Autodesk Inventor part; units mm, degrees
(part 2 of 2)
sketch "PCB草图" plane through (0, 3.5, 0) normal (0, 1, 0) x (1, 0, 0)
  line L0 (-85.025, -120.975) -> (-85.025, -135.025) projected
  line L1 (-85.025, -135.025) -> (-70.975, -135.025) projected
  line L2 (-70.975, -120.975) -> (-85.025, -120.975) projected
  line L3 (-70.975, -135.025) -> (-70.975, -120.975) projected
  line L4 (-85.025, -135.025) -> (-70.975, -120.975) construction
  line L5 (-70.975, -135.025) -> (-85.025, -120.975) construction
  line L6 (-85.025, -116.025) -> (-70.975, -116.025) projected
  line L7 (-85.025, -101.975) -> (-85.025, -116.025) projected
  line L8 (-70.975, -101.975) -> (-85.025, -101.975) projected
  line L9 (-70.975, -116.025) -> (-70.975, -101.975) projected
  line L10 (-85.025, -116.025) -> (-70.975, -101.975) construction
  line L11 (-70.975, -116.025) -> (-85.025, -101.975) construction
  line L12 (-85.025, -82.975) -> (-85.025, -97.025) projected
  line L13 (-85.025, -97.025) -> (-70.975, -97.025) projected
  line L14 (-70.975, -97.025) -> (-70.975, -82.975) projected
  line L15 (-70.975, -82.975) -> (-85.025, -82.975) projected
  line L16 (-85.025, -97.025) -> (-70.975, -82.975) construction
  line L17 (-70.975, -97.025) -> (-85.025, -82.975) construction
  line L18 (-85.025, -78.025) -> (-70.975, -78.025) projected
  line L19 (-85.025, -63.975) -> (-85.025, -78.025) projected
  line L20 (-70.975, -63.975) -> (-85.025, -63.975) projected
  line L21 (-70.975, -78.025) -> (-70.975, -63.975) projected
  line L22 (-85.025, -78.025) -> (-70.975, -63.975) construction
  line L23 (-70.975, -78.025) -> (-85.025, -63.975) construction
  line L24 (-51.0903, -48.4209) -> (-51.0903, -62.4709) projected
  line L25 (-51.0903, -62.4709) -> (-37.0403, -62.4709) projected
  line L26 (-37.0403, -62.4709) -> (-37.0403, -48.4209) projected
  line L27 (-37.0403, -48.4209) -> (-51.0903, -48.4209) projected
  line L28 (-51.0903, -62.4709) -> (-37.0403, -48.4209) construction
  line L29 (-37.0403, -62.4709) -> (-51.0903, -48.4209) construction
  line L30 (-47.0095, -25.2779) -> (-47.0095, -39.3279) projected
  line L31 (-47.0095, -39.3279) -> (-32.9595, -39.3279) projected
  line L32 (-32.9595, -25.2779) -> (-47.0095, -25.2779) projected
  line L33 (-32.9595, -39.3279) -> (-32.9595, -25.2779) projected
  line L34 (-47.0095, -39.3279) -> (-32.9595, -25.2779) construction
  line L35 (-32.9595, -39.3279) -> (-47.0095, -25.2779) construction
  line L36 (-33.5305, -6.0279) -> (-33.5305, -20.0779) projected
  line L37 (-33.5305, -20.0779) -> (-19.4805, -20.0779) projected
  line L38 (-19.4805, -6.0279) -> (-33.5305, -6.0279) projected
  line L39 (-19.4805, -20.0779) -> (-19.4805, -6.0279) projected
  line L40 (-33.5305, -20.0779) -> (-19.4805, -6.0279) construction
  line L41 (-19.4805, -20.0779) -> (-33.5305, -6.0279) construction
  line L42 (-78.6994, 7.7892) -> (-78.6994, -6.2608) projected
  line L43 (-78.6994, -6.2608) -> (-64.6494, -6.2608) projected
  line L44 (-64.6494, 7.7892) -> (-78.6994, 7.7892) projected
  line L45 (-64.6494, -6.2608) -> (-64.6494, 7.7892) projected
  line L46 (-78.6994, -6.2608) -> (-64.6494, 7.7892) construction
  line L47 (-64.6494, -6.2608) -> (-78.6994, 7.7892) construction
  line L48 (-53.7945, 9.9681) -> (-53.7945, -4.0819) projected
  line L49 (-53.7945, -4.0819) -> (-39.7445, -4.0819) projected
  line L50 (-39.7445, 9.9681) -> (-53.7945, 9.9681) projected
  line L51 (-39.7445, -4.0819) -> (-39.7445, 9.9681) projected
  line L52 (-53.7945, -4.0819) -> (-39.7445, 9.9681) construction
  line L53 (-39.7445, -4.0819) -> (-53.7945, 9.9681) construction
  line L54 (-31.3662, 20.7099) -> (-31.3662, 6.6599) projected
  line L55 (-31.3662, 6.6599) -> (-17.3162, 6.6599) projected
  line L56 (-17.3162, 6.6599) -> (-17.3162, 20.7099) projected
  line L57 (-17.3162, 20.7099) -> (-31.3662, 20.7099) projected
  line L58 (-31.3662, 6.6599) -> (-17.3162, 20.7099) construction
  line L59 (-17.3162, 6.6599) -> (-31.3662, 20.7099) construction
  line L60 (-54.0839, 16.3969) -> (-54.0839, 30.4469) projected
  line L61 (-54.0839, 30.4469) -> (-68.1339, 30.4469) projected
  line L62 (-68.1339, 30.4469) -> (-68.1339, 16.3969) projected
  line L63 (-68.1339, 16.3969) -> (-54.0839, 16.3969) projected
  line L64 (-68.1339, 16.3969) -> (-54.0839, 30.4469) construction
  line L65 (-54.0839, 16.3969) -> (-68.1339, 30.4469) construction
  line L66 (-45.7056, 41.1887) -> (-45.7056, 27.1387) projected
  line L67 (-45.7056, 27.1387) -> (-31.6556, 27.1387) projected
  line L68 (-31.6556, 27.1387) -> (-31.6556, 41.1887) projected
  line L69 (-31.6556, 41.1887) -> (-45.7056, 41.1887) projected
  line L70 (-45.7056, 27.1387) -> (-31.6556, 41.1887) construction
  line L71 (-31.6556, 27.1387) -> (-45.7056, 41.1887) construction
  line L72 (-62.6344, 39.8892) -> (-62.6344, 53.9392) projected
  line L73 (-76.6844, 39.8892) -> (-62.6344, 39.8892) projected
  line L74 (-76.6844, 53.9392) -> (-76.6844, 39.8892) projected
  line L75 (-62.6344, 53.9392) -> (-76.6844, 53.9392) projected
  line L76 (-62.6344, 39.8892) -> (-76.6844, 53.9392) construction
  line L77 (-76.6844, 39.8892) -> (-62.6344, 53.9392) construction
  line L78 (-78.8633, 64.7941) -> (-64.8133, 64.7941) projected
  line L79 (-78.8633, 78.8441) -> (-78.8633, 64.7941) projected
  line L80 (-64.8133, 78.8441) -> (-78.8633, 78.8441) projected
  line L81 (-64.8133, 64.7941) -> (-64.8133, 78.8441) projected
  line L82 (-78.8633, 64.7941) -> (-64.8133, 78.8441) construction
  line L83 (-64.8133, 64.7941) -> (-78.8633, 78.8441) construction
  line L84 (-56.435, 89.5859) -> (-56.435, 75.5359) projected
  line L85 (-56.435, 75.5359) -> (-42.385, 75.5359) projected
  line L86 (-42.385, 75.5359) -> (-42.385, 89.5859) projected
  line L87 (-42.385, 89.5859) -> (-56.435, 89.5859) projected
  line L88 (-56.435, 75.5359) -> (-42.385, 89.5859) construction
  line L89 (-42.385, 75.5359) -> (-56.435, 89.5859) construction
  line L90 (12.8421, -27.1872) -> (12.8421, -41.2372) projected
  line L91 (12.8421, -41.2372) -> (26.8921, -41.2372) projected
  line L92 (26.8921, -41.2372) -> (26.8921, -27.1872) projected
  line L93 (26.8921, -27.1872) -> (12.8421, -27.1872) projected
  line L94 (12.8421, -41.2372) -> (26.8921, -27.1872) construction
  line L95 (26.8921, -41.2372) -> (12.8421, -27.1872) construction
  line L96 (19.8671, -0.128) -> (19.8671, -14.178) projected
  line L97 (19.8671, -14.178) -> (33.9171, -14.178) projected
  line L98 (33.9171, -14.178) -> (33.9171, -0.128) projected
  line L99 (33.9171, -0.128) -> (19.8671, -0.128) projected
  line L100 (19.8671, -14.178) -> (33.9171, -0.128) construction
  line L101 (33.9171, -14.178) -> (19.8671, -0.128) construction
  line L102 (12.8421, 12.8811) -> (26.8921, 12.8811) projected
  line L103 (12.8421, 26.9311) -> (12.8421, 12.8811) projected
  line L104 (26.8921, 26.9311) -> (12.8421, 26.9311) projected
  line L105 (26.8921, 12.8811) -> (26.8921, 26.9311) projected
  line L106 (12.8421, 12.8811) -> (26.8921, 26.9311) construction
  line L107 (26.8921, 12.8811) -> (12.8421, 26.9311) construction
  line L108 (6.4757, 37.0569) -> (20.5257, 37.0569) projected
  line L109 (6.4757, 51.1069) -> (6.4757, 37.0569) projected
  line L110 (20.5257, 51.1069) -> (6.4757, 51.1069) projected
  line L111 (20.5257, 37.0569) -> (20.5257, 51.1069) projected
  line L112 (6.4757, 37.0569) -> (20.5257, 51.1069) construction
  line L113 (20.5257, 37.0569) -> (6.4757, 51.1069) construction
  circle A0 centre (-40.4289, -130.4289) radius 1.5 projected
  circle A1 centre (4.4289, -130.4289) radius 1.5 projected
  circle A2 centre (44.4289, -44.4289) radius 1.35 projected
  circle A3 centre (-18.0001, -44.4289) radius 1.5 projected
  circle A4 centre (-80.4289, -44.4289) radius 1.5 projected
  circle A5 centre (-80.4289, 44.4289) radius 1.5 projected
  circle A6 centre (-18.0001, 44.4289) radius 1.5 projected
  circle A7 centre (44.4289, 44.4289) radius 1.5 projected
  circle A8 centre (-40.4289, 130.4289) radius 1.5 projected
  circle A9 centre (4.4289, 130.4289) radius 1.5 projected
  circle A10 centre (-93.9645, -10.9645) radius 1.5 projected
  circle A11 centre (-93.9645, 10.9645) radius 1.35 projected
  circle A12 centre (-93.9645, 65.5355) radius 1.35 projected
  circle A13 centre (-93.9645, 87.4645) radius 1.5 projected
  line L114 (-87.5, 91) -> (-97.5, 91)
  line L115 (-97.5, 91) -> (-97.5, 62)
  line L116 (-97.5, 62) -> (-87.5, 62)
  line L117 (-87.5, 62) -> (-87.5, 14.5)
  line L118 (-87.5, 14.5) -> (-97.5, 14.5)
  line L119 (-97.5, -14.5) -> (-97.5, 14.5)
  line L120 (-97.5, -14.5) -> (-87.5, -14.5)
  line L121 (-87.5, -14.5) -> (-87.5, -137.5)
  line L122 (-87.5, -137.5) -> (51.5, -137.5)
  line L123 (51.5, 137.5) -> (-87.5, 137.5)
  line L124 (-87.5, 137.5) -> (-87.5, 91)
  line L125 (-54.2561, 64.6811) -> (-54.2561, 50.6311) projected
  line L126 (-54.2561, 50.6311) -> (-40.2061, 50.6311) projected
  line L127 (-40.2061, 50.6311) -> (-40.2061, 64.6811) projected
  line L128 (-40.2061, 64.6811) -> (-54.2561, 64.6811) projected
  line L129 (-54.2561, 50.6311) -> (-40.2061, 64.6811) construction
  line L130 (-40.2061, 50.6311) -> (-54.2561, 64.6811) construction
  line L131 (51.5, 137.5) -> (31.5, 137.5)
  line L132 (31.5, 117.5) -> (51.5, 117.5)
  line L133 (31.5, 117.5) -> (-20.5, 117.5)
  line L134 (-20.5, 117.5) -> (-20.5, 95.5)
  line L135 (-20.5, 95.5) -> (31.5, 95.5)
  line L136 (31.5, 95.5) -> (31.5, 117.5)
  line L137 (51.5, 117.5) -> (51.5, 137.5)
  line L138 (31.5, 95.5) -> (31.5, 75.5)
  line L139 (31.5, 75.5) -> (51.5, 75.5)
  line L140 (51.5, 75.5) -> (51.5, 75.5359)
  line L141 (51.5, -117.5) -> (31.5, -117.5)
  line L142 (31.5, -117.5) -> (31.5, -97.5)
  line L143 (31.5, -97.5) -> (51.5, -97.5)
  line L144 (51.5, -137.5) -> (51.5, -117.5)
  line L145 (51.5, -97.5) -> (51.5, 75.5)
  point P0 (0, 0)
  dimension "d459" = 20
  dimension "d460" = 20
  dimension "d461" = 52
  dimension "d462" = 22
  dimension "d463" = 20
  dimension "d464" = 20
  dimension "d466" = 20
  dimension "d467" = 20
  constraints: 52 end point, 1 point on line
  measures "d459" distance of L132.end L132.start
  measures "d460" distance of L132.start L131.end
  measures "d461" distance of L135.end L134.end
  measures "d462" distance of L134.end L133.end
  measures "d463" distance of L139.end L138.end
  measures "d464" distance of L138.end L138.start
  measures "d466" distance of L142.end L143.end
  measures "d467" distance of L141.end L142.end
